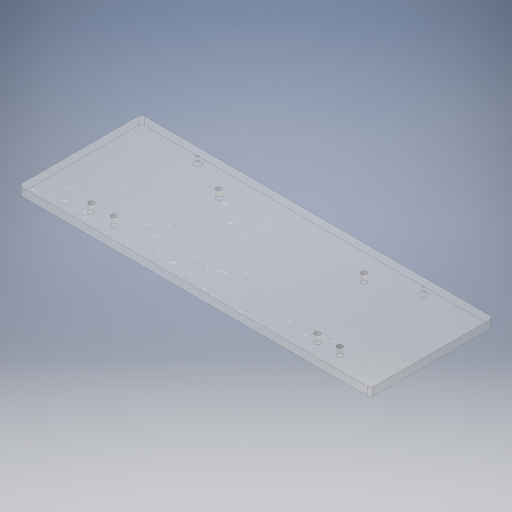
# Autodesk Inventor part: BT703_trajan20_21
Saved by Autodesk Inventor 2023 (Build 270158000, 158)
## iProperties
Company: HTBLA Kaindorf
RuleStatus: InUse
Created: 2022-08-21
Part Number: BT703_trajan20_21
Project: Zeichenmaschine_v2
Material: Acryl
Description: Plexitür_200x80
Document SubType Name: Modeling
Designer: trajan20
Density: 1.188 g/cm^3
Appearance: Transparent - farblos
Mass: 98.0589 g
Surface Area: 362.976 cm^2
Volume: 82.5412 cm^3
AfterDocNew0: iProperties-Editor_aufrufen
Author: jan
Keywords: 2021
Autodesk Inventor part; units mm, degrees
ref_plane "YZ Plane" through (0, 0, 0) normal (1, 0, 0) x (0, 1, 0)
ref_plane "XZ Plane" through (0, 0, 0) normal (0, 1, 0) x (-1, 0, 0)
derived "BT000_trajan20_22_Zeichenmaschine_neu_Masterskizze.ipt"
sketch "Skizze3" plane through (0, 0, 0) normal (0, 0, 1) x (1, 0, 0)
  line L0 (0, 0) -> (-76, 0)
  line L1 (-76, 0) -> (-76, 218)
  line L2 (-76, 218) -> (0, 218)
  line L3 (0, 218) -> (0, 0)
  point P0 (-13, 186)
  point P1 (-13, 172)
  point P2 (-71.81, 179)
  point P3 (-60, 154)
  point P4 (-76, 109)
  dimension "d4" = 218
  dimension "d5" = 76
  dimension "d9" = 32
  dimension "d13" = 71.81
  dimension "d14" = 39
  dimension "d15" = 60
  dimension "d32" = 14
  dimension "d33" = 13
  dimension "d34" = 45
  constraints: 8 end point, 2 parallel, 1 horizontal, 1 midpoint, 1 perpendicular, 1 vertical alignment
  measures "d4" distance between parallel lines of L0 L2
  measures "d5" distance between parallel lines of L1 L3
  measures "d9" distance from line of point (-13, 186) L2
  measures "d13" distance from line of L3 point (-71.81, 179)
  measures "d14" distance from line of L2 point (-71.81, 179)
  measures "d15" distance from line of L3 point (-60, 154)
  measures "d32" distance of point (-13, 186) point (-13, 172)
  measures "d33" distance from line of point (-13, 172) L3
  measures "d34" vertical distance of point (-76, 109) point (-60, 154)
extrude "Extrusion3" add sketch "Skizze3" along normal blind 5
fillet "Rundung1" radius 2 4 edges at (0, 218, 2.5) (-76, 218, 2.5) (-76, 0, 2.5) (0, 0, 2.5)
ref_plane "Arbeitsebene1" through (-76, 109, 0) normal (0, -1, 0) x (1, 0, 0)
hole "Bohrung1" at (-13, 186, 0) at (-13, 172, 0) at (-60, 154, 0) direction (0, 0, 1) diameter 3.242 end through all thread size "M4x0.7" class "6H" standard "ISO Metric profile"
hole "Bohrung2" at (-71.81, 179, 0) direction (0, 0, 1) diameter 1.567 depth 4.2 tip angle 118 countersink diameter 4.5 countersink angle 90 thread size "M2x0.4" class "6H" standard "ISO Metric profile"
mirror "Spiegeln1" about plane through (-76, 109, 0) normal (0, -1, 0) of "Bohrung2", "Bohrung1"
